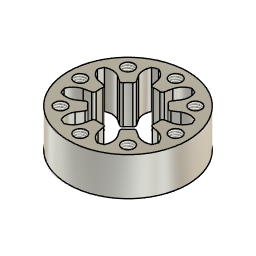
[J,L]C-578VA Joint (Autodesk Fusion 360 design; units mm, degrees)
Autodesk Fusion 360 part; units mm, degrees
sketch "スケッチ1" plane through (0, 0, 0) normal (0, 0, 1) x (1, 0, 0)
  arc A0 (4.7176, 3.7073) -> (3.7073, 4.7176) centre (0, 0) ccw
  arc A1 (0.7144, 5.9573) -> (1.2643, 6.3562) centre (0.7739, 6.4538) ccw
  line L0 (1.5607, 7.8463) -> (1.2643, 6.3562)
  arc A2 (0.7144, 5.9573) -> (-0.7144, 5.9573) centre (0, 0) ccw
  line L1 (3.6005, 5.3885) -> (4.4446, 6.6518)
  arc A3 (9.9013, 3.495) -> (9.4726, 4.5299) centre (0, 0) ccw
  line L2 (7.8463, -1.5607) -> (6.3562, -1.2643)
  arc A4 (-0.7144, -5.9573) -> (-1.2643, -6.3562) centre (-0.7739, -6.4538) ccw
  arc A5 (4.4446, 6.6518) -> (4.5299, 9.4726) centre (1.841, 8.1423) ccw
  arc A6 (-6.6518, 4.4446) -> (-9.4726, 4.5299) centre (-8.1423, 1.841) ccw
  arc A7 (9.9013, -3.495) -> (7.8463, -1.5607) centre (7.0593, -4.4556) ccw
  arc A8 (6.6518, -4.4446) -> (9.4726, -4.5299) centre (8.1423, -1.841) ccw
  arc A9 (3.495, 9.9013) -> (1.5607, 7.8463) centre (4.4556, 7.0593) ccw
  arc A10 (7.8463, 1.5607) -> (9.9013, 3.495) centre (7.0593, 4.4556) ccw
  arc A11 (5.3885, -3.6005) -> (4.7176, -3.7073) centre (5.1108, -4.0162) ccw
  line L3 (-1.2643, 6.3562) -> (-1.5607, 7.8463)
  arc A12 (3.7073, -4.7176) -> (4.7176, -3.7073) centre (0, 0) ccw
  line L4 (-4.4446, 6.6518) -> (-3.6005, 5.3885)
  arc A13 (-4.7176, -3.7073) -> (-3.7073, -4.7176) centre (0, 0) ccw
  arc A14 (-4.7176, -3.7073) -> (-5.3885, -3.6005) centre (-5.1108, -4.0162) ccw
  arc A15 (4.5299, -9.4726) -> (4.4446, -6.6518) centre (1.841, -8.1423) ccw
  line L5 (6.3562, 1.2643) -> (7.8463, 1.5607)
  arc A16 (-5.3885, 3.6005) -> (-4.7176, 3.7073) centre (-5.1108, 4.0162) ccw
  arc A17 (-3.7073, 4.7176) -> (-3.6005, 5.3885) centre (-4.0162, 5.1108) ccw
  arc A18 (-3.6005, -5.3885) -> (-3.7073, -4.7176) centre (-4.0162, -5.1108) ccw
  arc A19 (3.495, -9.9013) -> (4.5299, -9.4726) centre (0, 0) ccw
  arc A20 (-5.9573, 0.7144) -> (-6.3562, 1.2643) centre (-6.4538, 0.7739) ccw
  arc A21 (4.5299, 9.4726) -> (3.495, 9.9013) centre (0, 0) ccw
  arc A22 (5.9573, -0.7144) -> (5.9573, 0.7144) centre (0, 0) ccw
  arc A23 (9.4726, -4.5299) -> (9.9013, -3.495) centre (0, 0) ccw
  arc A24 (5.9573, -0.7144) -> (6.3562, -1.2643) centre (6.4538, -0.7739) ccw
  arc A25 (3.6005, 5.3885) -> (3.7073, 4.7176) centre (4.0162, 5.1108) ccw
  circle A26 centre (0, 0) radius 1
  arc A27 (-0.7144, -5.9573) -> (0.7144, -5.9573) centre (0, 0) ccw
  arc A28 (3.7073, -4.7176) -> (3.6005, -5.3885) centre (4.0162, -5.1108) ccw
  arc A29 (-3.495, 9.9013) -> (-4.5299, 9.4726) centre (0, 0) ccw
  arc A30 (-1.2643, 6.3562) -> (-0.7144, 5.9573) centre (-0.7739, 6.4538) ccw
  arc A31 (4.7176, 3.7073) -> (5.3885, 3.6005) centre (5.1108, 4.0162) ccw
  arc A32 (-1.5607, 7.8463) -> (-3.495, 9.9013) centre (-4.4556, 7.0593) ccw
  arc A33 (-4.5299, 9.4726) -> (-4.4446, 6.6518) centre (-1.841, 8.1423) ccw
  arc A34 (1.5607, -7.8463) -> (3.495, -9.9013) centre (4.4556, -7.0593) ccw
  arc A35 (-9.4726, 4.5299) -> (-9.9013, 3.495) centre (0, 0) ccw
  arc A36 (-9.9013, 3.495) -> (-7.8463, 1.5607) centre (-7.0593, 4.4556) ccw
  line L6 (-5.3885, 3.6005) -> (-6.6518, 4.4446)
  arc A37 (-3.7073, 4.7176) -> (-4.7176, 3.7073) centre (0, 0) ccw
  arc A38 (-4.4446, -6.6518) -> (-4.5299, -9.4726) centre (-1.841, -8.1423) ccw
  line L7 (-6.3562, -1.2643) -> (-7.8463, -1.5607)
  line L8 (1.2643, -6.3562) -> (1.5607, -7.8463)
  line L9 (4.4446, -6.6518) -> (3.6005, -5.3885)
  arc A39 (-9.4726, -4.5299) -> (-6.6518, -4.4446) centre (-8.1423, -1.841) ccw
  arc A40 (1.2643, -6.3562) -> (0.7144, -5.9573) centre (0.7739, -6.4538) ccw
  line L10 (6.6518, 4.4446) -> (5.3885, 3.6005)
  arc A41 (-4.5299, -9.4726) -> (-3.495, -9.9013) centre (0, 0) ccw
  arc A42 (6.3562, 1.2643) -> (5.9573, 0.7144) centre (6.4538, 0.7739) ccw
  line L11 (5.3885, -3.6005) -> (6.6518, -4.4446)
  arc A43 (9.4726, 4.5299) -> (6.6518, 4.4446) centre (8.1423, 1.841) ccw
  line L12 (-7.8463, 1.5607) -> (-6.3562, 1.2643)
  arc A44 (-3.495, -9.9013) -> (-1.5607, -7.8463) centre (-4.4556, -7.0593) ccw
  line L13 (-1.5607, -7.8463) -> (-1.2643, -6.3562)
  arc A45 (-9.9013, -3.495) -> (-9.4726, -4.5299) centre (0, 0) ccw
  line L14 (-3.6005, -5.3885) -> (-4.4446, -6.6518)
  arc A46 (-7.8463, -1.5607) -> (-9.9013, -3.495) centre (-7.0593, -4.4556) ccw
  line L15 (-6.6518, -4.4446) -> (-5.3885, -3.6005)
  arc A47 (-5.9573, 0.7144) -> (-5.9573, -0.7144) centre (0, 0) ccw
  arc A48 (-6.3562, -1.2643) -> (-5.9573, -0.7144) centre (-6.4538, -0.7739) ccw
  circle A49 centre (0, 0) radius 12.5
  dimension "d1" = 25
  constraint coincident A0.centre A2.centre
  measures "d1" diameter of A49
extrude "押し出し1" add sketch "スケッチ1" along normal blind 8 contours A49
sketch "スケッチ2" plane through (0, 0, 8) normal (0, 0, 1) x (-1, 0, 0)
  arc A0 (7.8463, 1.5607) -> (9.9013, 3.495) centre (7.0593, 4.4556) ccw
  line L0 (7.8463, 1.5607) -> (6.3562, 1.2643)
  arc A1 (6.3562, 1.2643) -> (5.9573, 0.7144) centre (6.4538, 0.7739) ccw
  arc A2 (5.9573, -0.7144) -> (5.9573, 0.7144) centre (0, 0) ccw
  arc A3 (5.9573, -0.7144) -> (6.3562, -1.2643) centre (6.4538, -0.7739) ccw
  line L1 (6.3562, -1.2643) -> (7.8463, -1.5607)
  arc A4 (9.9013, -3.495) -> (7.8463, -1.5607) centre (7.0593, -4.4556) ccw
  arc A5 (9.4726, -4.5299) -> (9.9013, -3.495) centre (0, 0) ccw
  arc A6 (6.6518, -4.4446) -> (9.4726, -4.5299) centre (8.1423, -1.841) ccw
  line L2 (6.6518, -4.4446) -> (5.3885, -3.6005)
  arc A7 (5.3885, -3.6005) -> (4.7176, -3.7073) centre (5.1108, -4.0162) ccw
  arc A8 (3.7073, -4.7176) -> (4.7176, -3.7073) centre (0, 0) ccw
  arc A9 (3.7073, -4.7176) -> (3.6005, -5.3885) centre (4.0162, -5.1108) ccw
  line L3 (3.6005, -5.3885) -> (4.4446, -6.6518)
  arc A10 (4.5299, -9.4726) -> (4.4446, -6.6518) centre (1.841, -8.1423) ccw
  arc A11 (3.495, -9.9013) -> (4.5299, -9.4726) centre (0, 0) ccw
  arc A12 (1.5607, -7.8463) -> (3.495, -9.9013) centre (4.4556, -7.0593) ccw
  line L4 (1.5607, -7.8463) -> (1.2643, -6.3562)
  arc A13 (1.2643, -6.3562) -> (0.7144, -5.9573) centre (0.7739, -6.4538) ccw
  arc A14 (-0.7144, -5.9573) -> (0.7144, -5.9573) centre (0, 0) ccw
  arc A15 (-0.7144, -5.9573) -> (-1.2643, -6.3562) centre (-0.7739, -6.4538) ccw
  line L5 (-1.2643, -6.3562) -> (-1.5607, -7.8463)
  arc A16 (-3.495, -9.9013) -> (-1.5607, -7.8463) centre (-4.4556, -7.0593) ccw
  arc A17 (-4.5299, -9.4726) -> (-3.495, -9.9013) centre (0, 0) ccw
  arc A18 (-4.4446, -6.6518) -> (-4.5299, -9.4726) centre (-1.841, -8.1423) ccw
  line L6 (-4.4446, -6.6518) -> (-3.6005, -5.3885)
  arc A19 (-3.6005, -5.3885) -> (-3.7073, -4.7176) centre (-4.0162, -5.1108) ccw
  arc A20 (-4.7176, -3.7073) -> (-3.7073, -4.7176) centre (0, 0) ccw
  arc A21 (-4.7176, -3.7073) -> (-5.3885, -3.6005) centre (-5.1108, -4.0162) ccw
  line L7 (-5.3885, -3.6005) -> (-6.6518, -4.4446)
  arc A22 (-9.4726, -4.5299) -> (-6.6518, -4.4446) centre (-8.1423, -1.841) ccw
  arc A23 (-9.9013, -3.495) -> (-9.4726, -4.5299) centre (0, 0) ccw
  arc A24 (-7.8463, -1.5607) -> (-9.9013, -3.495) centre (-7.0593, -4.4556) ccw
  line L8 (-7.8463, -1.5607) -> (-6.3562, -1.2643)
  arc A25 (-6.3562, -1.2643) -> (-5.9573, -0.7144) centre (-6.4538, -0.7739) ccw
  arc A26 (-5.9573, 0.7144) -> (-5.9573, -0.7144) centre (0, 0) ccw
  arc A27 (-5.9573, 0.7144) -> (-6.3562, 1.2643) centre (-6.4538, 0.7739) ccw
  line L9 (-6.3562, 1.2643) -> (-7.8463, 1.5607)
  arc A28 (-9.9013, 3.495) -> (-7.8463, 1.5607) centre (-7.0593, 4.4556) ccw
  arc A29 (-9.4726, 4.5299) -> (-9.9013, 3.495) centre (0, 0) ccw
  arc A30 (-6.6518, 4.4446) -> (-9.4726, 4.5299) centre (-8.1423, 1.841) ccw
  line L10 (-6.6518, 4.4446) -> (-5.3885, 3.6005)
  arc A31 (-5.3885, 3.6005) -> (-4.7176, 3.7073) centre (-5.1108, 4.0162) ccw
  arc A32 (-3.7073, 4.7176) -> (-4.7176, 3.7073) centre (0, 0) ccw
  arc A33 (-3.7073, 4.7176) -> (-3.6005, 5.3885) centre (-4.0162, 5.1108) ccw
  line L11 (-3.6005, 5.3885) -> (-4.4446, 6.6518)
  arc A34 (-4.5299, 9.4726) -> (-4.4446, 6.6518) centre (-1.841, 8.1423) ccw
  arc A35 (-3.495, 9.9013) -> (-4.5299, 9.4726) centre (0, 0) ccw
  arc A36 (-1.5607, 7.8463) -> (-3.495, 9.9013) centre (-4.4556, 7.0593) ccw
  line L12 (-1.5607, 7.8463) -> (-1.2643, 6.3562)
  arc A37 (-1.2643, 6.3562) -> (-0.7144, 5.9573) centre (-0.7739, 6.4538) ccw
  arc A38 (0.7144, 5.9573) -> (-0.7144, 5.9573) centre (0, 0) ccw
  arc A39 (0.7144, 5.9573) -> (1.2643, 6.3562) centre (0.7739, 6.4538) ccw
  line L13 (1.2643, 6.3562) -> (1.5607, 7.8463)
  arc A40 (3.495, 9.9013) -> (1.5607, 7.8463) centre (4.4556, 7.0593) ccw
  arc A41 (4.5299, 9.4726) -> (3.495, 9.9013) centre (0, 0) ccw
  arc A42 (4.4446, 6.6518) -> (4.5299, 9.4726) centre (1.841, 8.1423) ccw
  line L14 (4.4446, 6.6518) -> (3.6005, 5.3885)
  arc A43 (3.6005, 5.3885) -> (3.7073, 4.7176) centre (4.0162, 5.1108) ccw
  arc A44 (4.7176, 3.7073) -> (3.7073, 4.7176) centre (0, 0) ccw
  arc A45 (4.7176, 3.7073) -> (5.3885, 3.6005) centre (5.1108, 4.0162) ccw
  line L15 (5.3885, 3.6005) -> (6.6518, 4.4446)
  arc A46 (9.4726, 4.5299) -> (6.6518, 4.4446) centre (8.1423, 1.841) ccw
  arc A47 (9.9013, 3.495) -> (9.4726, 4.5299) centre (0, 0) ccw
  circle A48 centre (0, 0) radius 12.5
  line L16 (0, 0) -> (12.5, 0)
  line L17 (0, 0) -> (0, -12.5)
  line L18 (0, 0) -> (-12.5, 0)
  line L19 (0, 0) -> (0, 12.5)
  line L20 (0, 0) -> (-8.8388, -8.8388)
  line L21 (0, 0) -> (8.8388, -8.8388)
  line L22 (0, 0) -> (-8.8388, 8.8388)
  line L23 (0, 0) -> (8.8388, 8.8388)
  line L24 (8.8388, -8.8388) -> (7.0711, -7.0711)
  circle A49 centre (7.0711, -7.0711) radius 1.25
  circle A50 centre (10, 0) radius 1.25
  circle A51 centre (7.0711, 7.0711) radius 1.25
  circle A52 centre (0, 10) radius 1.25
  circle A53 centre (-7.0711, 7.0711) radius 1.25
  circle A54 centre (-10, 0) radius 1.25
  circle A55 centre (-7.0711, -7.0711) radius 1.25
  circle A56 centre (0, -10) radius 1.25
  dimension "d4" = 45
  dimension "d5" = 2.5
  dimension "d6" = 2.5
  dimension "d8" = 360
  constraint coincident A2.centre A5.centre
  constraint coincident A48 L16.end
  constraint horizontal L16
  constraint coincident A48 L17.end
  constraint perpendicular L16 L17
  constraint coincident A48 L18.end
  constraint perpendicular L17 L18
  constraint coincident A48 L19.end
  constraint perpendicular L16 L19
  constraint coincident A48 L20.end
  constraint coincident A48 L21.end
  constraint perpendicular L20 L21
  constraint coincident A48 L22.end
  constraint perpendicular L20 L22
  constraint coincident A48 L23.end
  constraint perpendicular L22 L23
  constraint parallel L21 L24
  constraint coincident L24.end A49.centre
  measures "d4" angle of L19 L20
  measures "d5" distance of L21.end L24.end
  measures "d6" diameter of A49
extrude "押し出し2" cut sketch "スケッチ2" against normal blind 8 contours L16 A50 | L16 A50 | L17 A56 | L17 A56 | L18 A54 | L18 A54 | L19 A52 | L19 A52 | L20 A55 | L20 A55 | L21 L24 A49 | L21 L24 A49 | L22 A53 | L22 A53 | L23 A51 | L23 A51
thread "ねじ1" "ISO Metric profile 3.0 M3x0.5 6H" major diameter 3.086 minor diameter 2.529 pitch 0.5 angle 60 resizes the face on face at (-11.2484, 0.0623, 2.6667)
thread "ねじ2" "ISO Metric profile 3.0 M3x0.5 6H" major diameter 3.086 minor diameter 2.529 pitch 0.5 angle 60 resizes the face on face at (-8.3149, 7.1955, 2.6667)
thread "ねじ3" "ISO Metric profile 3.0 M3x0.5 6H" major diameter 3.086 minor diameter 2.529 pitch 0.5 angle 60 resizes the face on face at (-1.2438, 10.1245, 2.6667)
thread "ねじ4" "ISO Metric profile 3.0 M3x0.5 6H" major diameter 3.086 minor diameter 2.529 pitch 0.5 angle 60 resizes the face on face at (5.8273, 7.1955, 2.6667)
thread "ねじ5" "ISO Metric profile 3.0 M3x0.5 6H" major diameter 3.086 minor diameter 2.529 pitch 0.5 angle 60 resizes the face on face at (8.7562, 0.1245, 2.6667)
thread "ねじ6" "ISO Metric profile 3.0 M3x0.5 6H" major diameter 3.086 minor diameter 2.529 pitch 0.5 angle 60 resizes the face on face at (5.8273, -6.9466, 2.6667)
thread "ねじ7" "ISO Metric profile 3.0 M3x0.5 6H" major diameter 3.086 minor diameter 2.529 pitch 0.5 angle 60 resizes the face on face at (-1.2438, -9.8755, 2.6667)
thread "ねじ8" "ISO Metric profile 3.0 M3x0.5 6H" major diameter 3.086 minor diameter 2.529 pitch 0.5 angle 60 resizes the face on face at (-8.3149, -6.9466, 2.6667)
